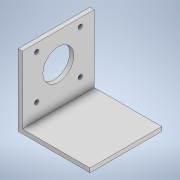
# Autodesk Inventor part: Metal_AttachmentBracket
Saved by Autodesk Inventor 2022 (Build 260153000, 153)
## iProperties
Created: 2022-02-26
Part Number: Metal_AttachmentBracket
Material: Generic
Document SubType Name: Modeling
Designer: Mlees
Density: 1 g/cm^3
Appearance: Default
Author: Mlees
Autodesk Inventor part; units mm, degrees
ref_plane "YZ Plane" through (0, 0, 0) normal (1, 0, 0) x (0, 1, 0)
ref_plane "XZ Plane" through (0, 0, 0) normal (0, 1, 0) x (-1, 0, 0)
ref_plane "XY Plane" through (0, 0, 0) normal (0, 0, 1) x (1, 0, 0)
sketch "Sketch1" plane through (0, 0, 0) normal (0, 0, 1) x (1, 0, 0)
  line L0 (0, 0) -> (0, 51)
  line L1 (0, 51) -> (3, 51)
  line L2 (3, 51) -> (3, 3)
  line L3 (3, 3) -> (51, 3)
  line L4 (51, 3) -> (51, 0)
  line L5 (51, 0) -> (0, 0)
  dimension "d0" = 51
  dimension "d1" = 3
  dimension "d2" = 48
  dimension "d3" = 48
  constraints: 12 end point, 5 perpendicular, 1 vertical
  measures "d0" distance of L0.start L0.end
  measures "d1" distance of L0.end L1.end
  measures "d2" distance of L1.end L2.end
  measures "d3" distance of L2.end L3.end
extrude "Extrusion1" add sketch "Sketch1" along normal blind 51
sketch "Sketch2" plane through (3, 3, 0) normal (1, 0, 0) x (0, 0, -1)
  line L0 (0, 48) -> (-51, 48) projected
  circle A0 centre (-25.5, 27) radius 11
  circle A1 centre (-41, 42.5) radius 1.5
  circle A2 centre (-10, 42.5) radius 1.5
  circle A3 centre (-10, 11.5) radius 1.5
  circle A4 centre (-41, 11.5) radius 1.5
  point P0 (0, -3)
  dimension "d7" = 22
  dimension "d12" = 3
  dimension "d13" = 3
  constraints: 5 centre point
  measures "d7" diameter of A0
  measures "d12" diameter of A1
  measures "d13" diameter of A2
extrude "Extrusion2" cut sketch "Sketch2" against normal up to surface (3 mm away)
body "Solid1"
